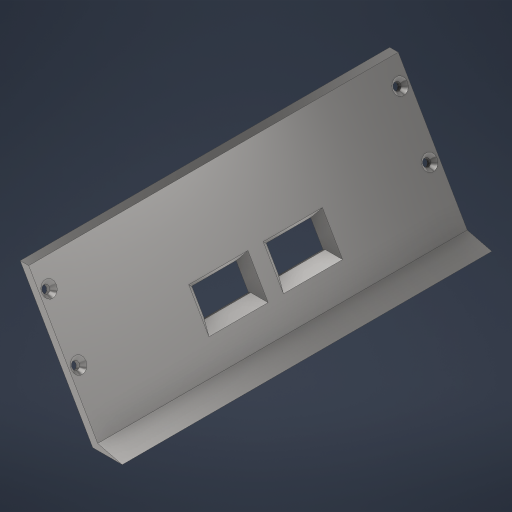
# Autodesk Inventor part: lemiesz
Saved by Autodesk Inventor 2024 (Build 280153000, 153)
## iProperties
Created: 2024-05-24
Part Number: lemiesz
Material: Steel
Document SubType Name: Modeling
Designer: Adam
Density: 7.85 g/cm^3
Appearance: Plate
Mass: 65.3515 g
Surface Area: 95.4294 cm^2
Volume: 8.32503 cm^3
Author: Adam
Autodesk Inventor part; units mm, degrees
ref_plane "YZ Plane" through (0, 0, 0) normal (1, 0, 0) x (0, 1, 0)
ref_plane "XZ Plane" through (0, 0, 0) normal (0, 1, 0) x (-1, 0, 0)
ref_plane "XY Plane" through (0, 0, 0) normal (0, 0, 1) x (1, 0, 0)
sketch "Sketch1" plane through (0, 0, 0) normal (0, 0, 1) x (1, 0, 0)
  line L0 (0, 0) -> (-8, 0)
  line L1 (-8, 0) -> (-27.6299, 34)
  line L2 (0, 0) -> (-6.6505, 1.6626)
  line L3 (-25.3205, 34) -> (-6.6505, 1.6626)
  line L4 (-27.6299, 34) -> (-25.3205, 34)
  dimension "d0" = 8
  dimension "d1" = 120
  dimension "d3" = 2
  constraints: 10 end point, 2 horizontal, 1 coincident, 1 parallel
  measures "d0" distance of L0.start L1.start
  measures "d1" angle of L0 L1
  measures "d3" distance between parallel lines of L3 L1
extrude "Extrusion1" add sketch "Sketch1" along normal mid plane 100
sketch "Sketch2" plane through (-25.3205, 34, 50) normal (0.8660254, 0.5, 0) x (0, 0, -1)
  line L0 (100, 0) -> (0, 0) projected
  point P0 (50, -42.1051)
  point P1 (2.5, -6)
  point P2 (2.5, -22)
  point P3 (97.5, -6)
  point P4 (97.5, -22)
hole "Hole1" at (-22.3205, 28.8038, 47.5) at (-14.3205, 14.9474, 47.5) at (-22.3205, 28.8038, -47.5) at (-14.3205, 14.9474, -47.5) direction (-0.8660254, -0.5, 0) diameter 2 end through all
chamfer "Chamfer1" distance 1 angle 45 4 edges at (-22.3205, 28.8038, 46.5) (-14.3205, 14.9474, 46.5) (-14.3205, 14.9474, -48.5) (-22.3205, 28.8038, -48.5) measured on face at (-22.3205, 28.8038, 46) measured on face at (-22.3205, 28.8038, -49) measured on face at (-14.3205, 14.9474, -49) measured on face at (-14.3205, 14.9474, 46)
sketch "Sketch6" plane through (0, 0, 0) normal (1, 0, 0) x (0, 1, 0)
  line L0 (1.6626, 50) -> (1.6626, -50) projected
  line L1 (15.6987, 14.2462) -> (9.6987, 14.2462)
  line L2 (9.6987, 14.2462) -> (9.6987, 2.2462)
  line L3 (9.6987, 2.2462) -> (15.6987, 2.2462)
  line L4 (15.6987, 2.2462) -> (15.6987, 14.2462)
  line L5 (15.6987, 14.2462) -> (9.6987, 2.2462) construction
  line L6 (9.6987, 14.2462) -> (15.6987, 2.2462) construction
  line L7 (15.6987, -5.9112) -> (9.6987, -5.9112)
  line L8 (9.6987, -5.9112) -> (9.6987, -17.9112)
  line L9 (9.6987, -17.9112) -> (15.6987, -17.9112)
  line L10 (15.6987, -17.9112) -> (15.6987, -5.9112)
  line L11 (15.6987, -5.9112) -> (9.6987, -17.9112) construction
  line L12 (9.6987, -5.9112) -> (15.6987, -17.9112) construction
  point P0 (0, 0)
  point P1 (34, 50)
  point P2 (34, 50)
  point P3 (12.6987, 8.2462)
  point P4 (12.6987, -11.9112)
  dimension "d22" = 6
  dimension "d23" = 12
  dimension "d24" = 6
  dimension "d25" = 12
  constraints: 24 end point, 4 midpoint, 4 parallel, 2 horizontal, 2 perpendicular
  measures "d22" distance of L3.end L2.end
  measures "d23" distance of L2.end L1.end
  measures "d24" distance of L9.end L8.end
  measures "d25" distance of L8.end L7.end
extrude "Extrusion2" cut sketch "Sketch6" against normal through all
chamfer "Chamfer2" distance 2 distance2 2 8 edges at (-13.0222, 12.6987, 2.2462) (-14.7543, 15.6987, 8.2462) (-13.0222, 12.6987, 14.2462) (-11.2902, 9.6987, 8.2462) (-14.7543, 15.6987, -11.9112) (-13.0222, 12.6987, -5.9112) (-13.0222, 12.6987, -17.9112) (-11.2902, 9.6987, -11.9112) measured on face at (-11.0402, 9.2657, 8.2462) measured on face at (-13.0222, 12.6987, -5.4112) measured on face at (-13.0222, 12.6987, -18.4112) measured on face at (-15.0043, 16.1317, 8.2462) measured on face at (-13.0222, 12.6987, 1.7462) measured on face at (-13.0222, 12.6987, 14.7462) measured on face at (-11.0402, 9.2657, -11.9112) measured on face at (-15.0043, 16.1317, -11.9112)
body "Solid1"
